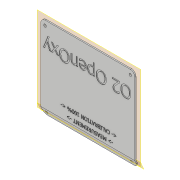
# Autodesk Inventor part: 03_Lid
Saved by Autodesk Inventor 2019.4 (Build 234330000, 330)
## iProperties
Created: 2021-06-05
Part Number: 03_Lid
Material: Generic
Document SubType Name: Modeling
Designer: diederichbenedict
Density: 1 g/cm^3
Appearance: Default
Author: diederichbenedict
Autodesk Inventor part; units mm, degrees
note: some values were not read from the file. Chosen so that the rebuilt part matches the saved one: sketch regions of "Extrusion1".
(part 1 of 2)
ref_plane "YZ Plane" through (0, 0, 0) normal (1, 0, 0) x (0, 1, 0)
ref_plane "XZ Plane" through (0, 0, 0) normal (0, 1, 0) x (-1, 0, 0)
ref_plane "XY Plane" through (0, 0, 0) normal (0, 0, 1) x (1, 0, 0)
ref_plane "Work Plane1" through (0, 0, 0) normal (0, 0, 1) x (1, 0, 0)
sketch "Sketch1" plane through (0, 0, 0) normal (0, 0, 1) x (1, 0, 0)
  ellipse E0 centre (-7.5, -84.2405) end of major axis (-7.5, -80.461) minor radius 1.5 projected
  ellipse E1 centre (-100.5, -84.2405) end of major axis (-100.5, -80.461) minor radius 1.5 projected
  ellipse E2 centre (-103, -7.7709) end of major axis (-103, -9.3506) minor radius 1.45 projected
  line L0 (-3, -61.2439) -> (-3, -12.7635) projected
  line L1 (-3, -61.2439) -> (-18, -61.2439) projected
  line L2 (-18, -90.5398) -> (-18, -61.2439) projected
  line L3 (0, -90.5398) -> (-18, -90.5398) projected
  line L4 (0, -7.7709) -> (0, -90.5398) projected
  ellipse E3 centre (-5, -7.7709) end of major axis (-5, -13.2183) minor radius 5 (0, -7.7709) -> (-5, -2.3235) ccw projected
  line L5 (-103, -2.3235) -> (-5, -2.3235) projected
  ellipse E4 centre (-103, -7.7709) end of major axis (-103, -13.2183) minor radius 5 (-103, -2.3235) -> (-108, -7.7709) ccw projected
  line L6 (-108, -90.5398) -> (-108, -7.7709) projected
  line L7 (-95, -90.5398) -> (-108, -90.5398) projected
  line L8 (-95, -61.2439) -> (-95, -90.5398) projected
  line L9 (-105, -61.2439) -> (-95, -61.2439) projected
  line L10 (-105, -12.7635) -> (-105, -61.2439) projected
  ellipse E5 centre (-103, -7.7709) end of major axis (-103, -13.2183) minor radius 5 (-105, -12.7635) -> (-98.4174, -5.5919) ccw projected
  line L11 (-9.5826, -5.5919) -> (-98.4174, -5.5919) projected
  ellipse E6 centre (-5, -7.7709) end of major axis (-5, -13.2183) minor radius 5 (-9.5826, -5.5919) -> (-3, -12.7635) ccw projected
  ellipse E7 centre (-5, -7.7709) end of major axis (-5, -9.3506) minor radius 1.45 projected
  line L12 (-18, -90.5398) -> (-95, -90.5398)
  point P0 (0, 0)
  constraints: 2 end point, 1 horizontal, 8 other
extrude "Extrusion1" add sketch "Sketch1" along normal blind 1.5 contours E0 | E1 | L1 L2 L12 L8 L9 L10 E5 L11 E6 L0 | L0 E6 L11 E5 L10 L9 L8 L7 L6 E4 L5 E3 L4 L3 L2 L1
ref_plane "Work Plane2" through (-54, -57.5226, 14.2761) normal (0, -0.3968725, 0.9178738) x (1, 0, 0)
sketch "Sketch2" plane through (-54, -57.5226, 14.2761) normal (0, -0.3968725, 0.9178738) x (1, 0, 0)
  circle A0 centre (49, -40) radius 1.45 projected
  circle A1 centre (-49, -40) radius 1.45 projected
  line L0 (-41, -35.9714) -> (-54, -35.9714) projected
  line L1 (-54, -40) -> (-54, -35.9714) projected
  arc A2 (-54, -40) -> (-49, -45) centre (-49, -40) ccw projected
  line L2 (49, -45) -> (-49, -45) projected
  arc A3 (49, -45) -> (54, -40) centre (49, -40) ccw projected
  line L3 (54, -35.9714) -> (54, -40) projected
  line L4 (54, -35.9714) -> (36, -35.9714) projected
  line L5 (36, -42) -> (36, -35.9714) projected
  line L6 (-41, -42) -> (36, -42) projected
  line L7 (-41, -35.9714) -> (-41, -42) projected
  line L8 (36, -35.9714) -> (-41, -35.9714)
  line L9 (-54, -35.9714) -> (54, -35.9714) projected
  line L10 (-54, 40) -> (-54, -35.9714) projected
  line L11 (54, -35.3761) -> (54, 40.5953) projected
  line L12 (-54, -35.9714) -> (54, -35.9714)
  line L13 (54, -35.9714) -> (54, -35.3761)
  line L14 (54, -35.3761) -> (-54, -35.3761)
  line L15 (-54, -35.3761) -> (-54, -35.9714)
  point P0 (54, 47.1327)
  constraints: 10 end point, 2 parallel, 1 collinear, 1 horizontal, 1 perpendicular
extrude "Extrusion2" add sketch "Sketch2" along normal up to surface (1.3768 mm away)
sketch "Sketch3" plane through (0, 0, 1.5) normal (0, 0, 1) x (1, 0, 0)
  ellipse E0 centre (-5, -7.7709) end of major axis (-5, -6.1911) minor radius 1.45 projected
  ellipse E1 centre (-103, -7.7709) end of major axis (-103, -6.1911) minor radius 1.45 projected
  line L0 (-108, -90.5398) -> (0, -90.5398) projected
  line L1 (0, -90.5398) -> (0, -7.7709) projected
  ellipse E2 centre (-5, -7.7709) end of major axis (-5, -13.2183) minor radius 5 (0, -7.7709) -> (-5, -2.3235) ccw projected
  line L2 (-5, -2.3235) -> (-103, -2.3235) projected
  ellipse E3 centre (-103, -7.7709) end of major axis (-103, -13.2183) minor radius 5 (-103, -2.3235) -> (-108, -7.7709) ccw projected
  line L3 (-108, -7.7709) -> (-108, -90.5398) projected
  line L4 (-3.7962, -33.7156) -> (-220.4518, -33.7156) construction
  line L5 (-220.4518, -33.7156) -> (-220.4518, 2.716) construction
  line L6 (-220.4518, 2.716) -> (-3.7962, 2.716) construction
  line L7 (-3.7962, 2.716) -> (-3.7962, -33.7156) construction
  line L8 (-24.8389, -87.8495) -> (-82.3672, -87.8495) construction
  line L9 (-82.3672, -87.8495) -> (-82.3672, -82.6215) construction
  line L10 (-82.3672, -82.6215) -> (-24.8389, -82.6215) construction
  line L11 (-24.8389, -82.6215) -> (-24.8389, -87.8495) construction
  line L12 (-20.6525, -79.3075) -> (-94.749, -79.3075) construction
  line L13 (-94.749, -79.3075) -> (-94.749, -72.5738) construction
  line L14 (-94.749, -72.5738) -> (-20.6525, -72.5738) construction
  line L15 (-20.6525, -72.5738) -> (-20.6525, -79.3075) construction
  spline S0 degree 2 poles (-14.4129, -31.9391) (-15.1575, -31.0668) (-15.9873, -28.5137) (-15.9873, -26.8754) knots 0 0 0 1 2 2 2
  spline S1 degree 2 poles (-15.9873, -26.8754) (-15.9873, -25.2798) (-15.1788, -22.6947) (-14.4129, -21.8224) knots 0 0 0 1 2 2 2
  spline S2 degree 2 poles (-14.4129, -21.8224) (-13.6044, -20.9076) (-11.4662, -20.0353) (-10.179, -20.0353) knots 0 0 0 1 2 2 2
  spline S3 degree 2 poles (-10.179, -20.0353) (-8.8492, -20.0353) (-6.7217, -20.9395) (-5.9451, -21.8224) knots 0 0 0 1 2 2 2
  spline S4 degree 2 poles (-5.9451, -21.8224) (-5.1898, -22.6947) (-4.3813, -25.2585) (-4.3813, -26.8754) knots 0 0 0 1 2 2 2
  spline S5 degree 2 poles (-4.3813, -26.8754) (-4.3813, -28.5243) (-5.2004, -31.0349) (-5.9557, -31.9391) knots 0 0 0 1 2 2 2
  spline S6 degree 2 poles (-5.9557, -31.9391) (-6.7217, -32.8114) (-8.8599, -33.7156) (-10.179, -33.7156) knots 0 0 0 1 2 2 2
  spline S7 degree 2 poles (-10.179, -33.7156) (-11.5194, -33.7156) (-13.6682, -32.7795) (-14.4129, -31.9391) knots 0 0 0 1 2 2 2
  spline S8 degree 2 poles (-14.1682, -26.8754) (-14.1682, -28.1733) (-13.6044, -30.1838) (-13.0938, -30.8434) knots 0 0 0 1 2 2 2
  spline S9 degree 2 poles (-13.0938, -30.8434) (-12.5725, -31.5242) (-11.1045, -32.205) (-10.1896, -32.205) knots 0 0 0 1 2 2 2
  spline S10 degree 2 poles (-10.1896, -32.205) (-9.2428, -32.205) (-7.8174, -31.5455) (-7.2748, -30.8434) knots 0 0 0 1 2 2 2
  spline S11 degree 2 poles (-7.2748, -30.8434) (-6.7536, -30.1732) (-6.2004, -28.152) (-6.2004, -26.8754) knots 0 0 0 1 2 2 2
  spline S12 degree 2 poles (-6.2004, -26.8754) (-6.2004, -24.2904) (-8.3705, -21.5458) (-10.1896, -21.5458) knots 0 0 0 1 2 2 2
  spline S13 degree 2 poles (-10.1896, -21.5458) (-12.0087, -21.5458) (-14.1682, -24.2904) (-14.1682, -26.8754) knots 0 0 0 1 2 2 2
  line L16 (-25.6252, -20.3118) -> (-17.5298, -20.3118)
  line L17 (-17.5298, -20.3118) -> (-17.5298, -22.1735)
  spline S14 degree 2 poles (-17.5298, -22.1735) (-18.4021, -22.9926) (-19.9552, -24.5138) (-20.6999, -25.3329) knots 0 0 0 1 2 2 2
  spline S15 degree 2 poles (-20.6999, -25.3329) (-22.1998, -26.9818) (-23.2955, -28.9605) (-23.2955, -30.0136) knots 0 0 0 1 2 2 2
  spline S16 degree 2 poles (-23.2955, -30.0136) (-23.2955, -30.5668) (-22.9551, -31.3966) (-22.6466, -31.6625) knots 0 0 0 1 2 2 2
  spline S17 degree 2 poles (-22.6466, -31.6625) (-22.3381, -31.9285) (-21.5296, -32.1944) (-21.0403, -32.1944) knots 0 0 0 1 2 2 2
  spline S18 degree 2 poles (-21.0403, -32.1944) (-20.5722, -32.1944) (-19.6148, -31.9604) (-19.1787, -31.7795) knots 0 0 0 1 2 2 2
  spline S19 degree 2 poles (-19.1787, -31.7795) (-18.8063, -31.6306) (-18.1149, -31.2051) (-17.9021, -31.0561) knots 0 0 0 1 2 2 2
  line L18 (-17.9021, -31.0561) -> (-17.8064, -31.0561)
  line L19 (-17.8064, -31.0561) -> (-17.8064, -32.9284)
  spline S20 degree 2 poles (-17.8064, -32.9284) (-18.3489, -33.1944) (-20.2956, -33.7156) (-21.168, -33.7156) knots 0 0 0 1 2 2 2
  spline S21 degree 2 poles (-21.168, -33.7156) (-23.0083, -33.7156) (-25.0827, -31.7689) (-25.0827, -30.1094) knots 0 0 0 1 2 2 2
  spline S22 degree 2 poles (-25.0827, -30.1094) (-25.0827, -29.3328) (-24.721, -28.035) (-24.4019, -27.4818) knots 0 0 0 1 2 2 2
  spline S23 degree 2 poles (-24.4019, -27.4818) (-24.0827, -26.9074) (-23.1572, -25.7797) (-22.6466, -25.2372) knots 0 0 0 1 2 2 2
  spline S24 degree 2 poles (-22.6466, -25.2372) (-21.8169, -24.333) (-19.785, -22.3969) (-19.1787, -21.8331) knots 0 0 0 1 2 2 2
  line L20 (-19.1787, -21.8331) -> (-25.6252, -21.8331)
  line L21 (-25.6252, -21.8331) -> (-25.6252, -20.3118)
  spline S25 degree 2 poles (-42.6778, -31.9391) (-43.4225, -31.0668) (-44.2523, -28.5137) (-44.2523, -26.8754) knots 0 0 0 1 2 2 2
  spline S26 degree 2 poles (-44.2523, -26.8754) (-44.2523, -25.2798) (-43.4438, -22.6947) (-42.6778, -21.8224) knots 0 0 0 1 2 2 2
  spline S27 degree 2 poles (-42.6778, -21.8224) (-41.8694, -20.9076) (-39.7311, -20.0353) (-38.4439, -20.0353) knots 0 0 0 1 2 2 2
  spline S28 degree 2 poles (-38.4439, -20.0353) (-37.1142, -20.0353) (-34.9866, -20.9395) (-34.2101, -21.8224) knots 0 0 0 1 2 2 2
  spline S29 degree 2 poles (-34.2101, -21.8224) (-33.4548, -22.6947) (-32.6463, -25.2585) (-32.6463, -26.8754) knots 0 0 0 1 2 2 2
  spline S30 degree 2 poles (-32.6463, -26.8754) (-32.6463, -28.5243) (-33.4654, -31.0349) (-34.2207, -31.9391) knots 0 0 0 1 2 2 2
  spline S31 degree 2 poles (-34.2207, -31.9391) (-34.9866, -32.8114) (-37.1248, -33.7156) (-38.4439, -33.7156) knots 0 0 0 1 2 2 2
  spline S32 degree 2 poles (-38.4439, -33.7156) (-39.7843, -33.7156) (-41.9332, -32.7795) (-42.6778, -31.9391) knots 0 0 0 1 2 2 2
  spline S33 degree 2 poles (-42.4332, -26.8754) (-42.4332, -28.1733) (-41.8694, -30.1838) (-41.3587, -30.8434) knots 0 0 0 1 2 2 2
  spline S34 degree 2 poles (-41.3587, -30.8434) (-40.8375, -31.5242) (-39.3694, -32.205) (-38.4546, -32.205) knots 0 0 0 1 2 2 2
  spline S35 degree 2 poles (-38.4546, -32.205) (-37.5078, -32.205) (-36.0823, -31.5455) (-35.5398, -30.8434) knots 0 0 0 1 2 2 2
  spline S36 degree 2 poles (-35.5398, -30.8434) (-35.0185, -30.1732) (-34.4654, -28.152) (-34.4654, -26.8754) knots 0 0 0 1 2 2 2
  spline S37 degree 2 poles (-34.4654, -26.8754) (-34.4654, -24.2904) (-36.6355, -21.5458) (-38.4546, -21.5458) knots 0 0 0 1 2 2 2
  spline S38 degree 2 poles (-38.4546, -21.5458) (-40.2737, -21.5458) (-42.4332, -24.2904) (-42.4332, -26.8754) knots 0 0 0 1 2 2 2
  spline S39 degree 2 poles (-54.2945, -25.5032) (-54.2945, -23.0352) (-51.9435, -20.1204) (-50.1457, -20.1204) knots 0 0 0 1 2 2 2
  spline S40 degree 2 poles (-50.1457, -20.1204) (-49.4116, -20.1204) (-48.284, -20.4608) (-47.6989, -20.8118) knots 0 0 0 1 2 2 2
  line L22 (-47.6989, -20.8118) -> (-47.6989, -16.6843)
  line L23 (-47.6989, -16.6843) -> (-46.0394, -16.6843)
  line L24 (-46.0394, -16.6843) -> (-46.0394, -30.1626)
  line L25 (-46.0394, -30.1626) -> (-47.6989, -30.1626)
  line L26 (-47.6989, -30.1626) -> (-47.6989, -29.1307)
  spline S41 degree 2 poles (-47.6989, -29.1307) (-48.3159, -29.6945) (-49.8265, -30.4391) (-50.7095, -30.4391) knots 0 0 0 1 2 2 2
  spline S42 degree 2 poles (-50.7095, -30.4391) (-52.4009, -30.4391) (-54.2945, -27.7584) (-54.2945, -25.5032) knots 0 0 0 1 2 2 2
  spline S43 degree 2 poles (-52.5817, -25.3117) (-52.5817, -27.0031) (-51.5073, -28.8647) (-50.3052, -28.8647) knots 0 0 0 1 2 2 2
  spline S44 degree 2 poles (-50.3052, -28.8647) (-49.6031, -28.8647) (-48.284, -28.2371) (-47.6989, -27.7478) knots 0 0 0 1 2 2 2
  line L27 (-47.6989, -27.7478) -> (-47.6989, -22.1522)
  spline S45 degree 2 poles (-47.6989, -22.1522) (-48.3479, -21.8437) (-49.2734, -21.6097) (-49.8691, -21.6097) knots 0 0 0 1 2 2 2
  spline S46 degree 2 poles (-49.8691, -21.6097) (-51.1563, -21.6097) (-52.5817, -23.5032) (-52.5817, -25.3117) knots 0 0 0 1 2 2 2
  spline S47 degree 2 poles (-60.2942, -20.0884) (-57.9326, -20.0884) (-55.337, -22.7373) (-55.337, -25.184) knots 0 0 0 1 2 2 2
  spline S48 degree 2 poles (-55.337, -25.184) (-55.337, -27.5882) (-57.8582, -30.4391) (-59.89, -30.4391) knots 0 0 0 1 2 2 2
  spline S49 degree 2 poles (-59.89, -30.4391) (-60.8049, -30.4391) (-62.2197, -29.9073) (-62.741, -29.3434) knots 0 0 0 1 2 2 2
  spline S50 degree 2 poles (-62.741, -29.3434) (-63.2729, -28.7796) (-63.8367, -27.152) (-63.8367, -25.9712) knots 0 0 0 1 2 2 2
  line L28 (-63.8367, -25.9712) -> (-63.8367, -25.067)
  line L29 (-63.8367, -25.067) -> (-57.0178, -25.067)
  spline S51 degree 2 poles (-57.0178, -25.067) (-57.0178, -23.3543) (-58.7411, -21.5352) (-60.273, -21.5352) knots 0 0 0 1 2 2 2
  spline S52 degree 2 poles (-60.273, -21.5352) (-60.8155, -21.5352) (-61.8687, -21.7799) (-62.2942, -21.9714) knots 0 0 0 1 2 2 2
  spline S53 degree 2 poles (-62.2942, -21.9714) (-62.741, -22.1841) (-63.358, -22.5564) (-63.5601, -22.7267) knots 0 0 0 1 2 2 2
  line L30 (-63.5601, -22.7267) -> (-63.6558, -22.7267)
  line L31 (-63.6558, -22.7267) -> (-63.6558, -20.9182)
  spline S54 degree 2 poles (-63.6558, -20.9182) (-63.3686, -20.8012) (-62.4963, -20.4608) (-62.1559, -20.365) knots 0 0 0 1 2 2 2
  spline S55 degree 2 poles (-62.1559, -20.365) (-61.6772, -20.2267) (-60.89, -20.0884) (-60.2942, -20.0884) knots 0 0 0 1 2 2 2
  spline S56 degree 2 poles (-62.2197, -26.3329) (-62.1984, -27.0031) (-61.9218, -27.9818) (-61.6559, -28.3116) knots 0 0 0 1 2 2 2
  spline S57 degree 2 poles (-61.6559, -28.3116) (-61.3687, -28.6839) (-60.4645, -29.0775) (-59.7943, -29.0775) knots 0 0 0 1 2 2 2
  spline S58 degree 2 poles (-59.7943, -29.0775) (-59.1347, -29.0775) (-58.2092, -28.6839) (-57.8262, -28.3009) knots 0 0 0 1 2 2 2
  spline S59 degree 2 poles (-57.8262, -28.3009) (-57.4539, -27.9073) (-57.071, -26.9605) (-57.0178, -26.3329) knots 0 0 0 1 2 2 2
  line L32 (-57.0178, -26.3329) -> (-62.2197, -26.3329)
  line L33 (-73.2512, -20.3118) -> (-71.5917, -20.3118)
  line L34 (-71.5917, -20.3118) -> (-71.5917, -25.9287)
  spline S60 degree 2 poles (-71.5917, -25.9287) (-71.5917, -26.6095) (-71.4641, -27.7797) (-71.2726, -28.1307) knots 0 0 0 1 2 2 2
  spline S61 degree 2 poles (-71.2726, -28.1307) (-71.0705, -28.503) (-70.3471, -28.8647) (-69.7301, -28.8647) knots 0 0 0 1 2 2 2
  spline S62 degree 2 poles (-69.7301, -28.8647) (-69.1131, -28.8647) (-67.8046, -28.2052) (-67.177, -27.6733) knots 0 0 0 1 2 2 2
  line L35 (-67.177, -27.6733) -> (-67.177, -20.3118)
  line L36 (-67.177, -20.3118) -> (-65.5175, -20.3118)
  line L37 (-65.5175, -20.3118) -> (-65.5175, -30.1626)
  line L38 (-65.5175, -30.1626) -> (-67.177, -30.1626)
  line L39 (-67.177, -30.1626) -> (-67.177, -29.0669)
  spline S63 degree 2 poles (-67.177, -29.0669) (-67.9216, -29.737) (-69.3578, -30.4391) (-70.1662, -30.4391) knots 0 0 0 1 2 2 2
  spline S64 degree 2 poles (-70.1662, -30.4391) (-71.613, -30.4391) (-73.2512, -28.5243) (-73.2512, -26.7052) knots 0 0 0 1 2 2 2
  line L40 (-73.2512, -26.7052) -> (-73.2512, -20.3118)
  spline S65 degree 2 poles (-84.9955, -31.9391) (-85.7402, -31.0668) (-86.5699, -28.5137) (-86.5699, -26.8754) knots 0 0 0 1 2 2 2
  spline S66 degree 2 poles (-86.5699, -26.8754) (-86.5699, -25.2798) (-85.7614, -22.6947) (-84.9955, -21.8224) knots 0 0 0 1 2 2 2
  spline S67 degree 2 poles (-84.9955, -21.8224) (-84.187, -20.9076) (-82.0488, -20.0353) (-80.7616, -20.0353) knots 0 0 0 1 2 2 2
  spline S68 degree 2 poles (-80.7616, -20.0353) (-79.4319, -20.0353) (-77.3043, -20.9395) (-76.5277, -21.8224) knots 0 0 0 1 2 2 2
  spline S69 degree 2 poles (-76.5277, -21.8224) (-75.7724, -22.6947) (-74.9639, -25.2585) (-74.9639, -26.8754) knots 0 0 0 1 2 2 2
  spline S70 degree 2 poles (-74.9639, -26.8754) (-74.9639, -28.5243) (-75.7831, -31.0349) (-76.5384, -31.9391) knots 0 0 0 1 2 2 2
  spline S71 degree 2 poles (-76.5384, -31.9391) (-77.3043, -32.8114) (-79.4425, -33.7156) (-80.7616, -33.7156) knots 0 0 0 1 2 2 2
  spline S72 degree 2 poles (-80.7616, -33.7156) (-82.102, -33.7156) (-84.2509, -32.7795) (-84.9955, -31.9391) knots 0 0 0 1 2 2 2
  spline S73 degree 2 poles (-84.7508, -26.8754) (-84.7508, -28.1733) (-84.187, -30.1838) (-83.6764, -30.8434) knots 0 0 0 1 2 2 2
  spline S74 degree 2 poles (-83.6764, -30.8434) (-83.1551, -31.5242) (-81.6871, -32.205) (-80.7723, -32.205) knots 0 0 0 1 2 2 2
  spline S75 degree 2 poles (-80.7723, -32.205) (-79.8255, -32.205) (-78.4, -31.5455) (-77.8575, -30.8434) knots 0 0 0 1 2 2 2
  spline S76 degree 2 poles (-77.8575, -30.8434) (-77.3362, -30.1732) (-76.783, -28.152) (-76.783, -26.8754) knots 0 0 0 1 2 2 2
  spline S77 degree 2 poles (-76.783, -26.8754) (-76.783, -24.2904) (-78.9532, -21.5458) (-80.7723, -21.5458) knots 0 0 0 1 2 2 2
  spline S78 degree 2 poles (-80.7723, -21.5458) (-82.5913, -21.5458) (-84.7508, -24.2904) (-84.7508, -26.8754) knots 0 0 0 1 2 2 2
  line L41 (-96.0058, -20.3118) -> (-93.9739, -20.3118)
  line L42 (-93.9739, -20.3118) -> (-91.5804, -24.0138)
  line L43 (-91.5804, -24.0138) -> (-89.123, -20.3118)
  line L44 (-89.123, -20.3118) -> (-87.2401, -20.3118)
  line L45 (-87.2401, -20.3118) -> (-90.6549, -25.1947)
  line L46 (-90.6549, -25.1947) -> (-87.272, -30.1626)
  line L47 (-87.272, -30.1626) -> (-89.3039, -30.1626)
  line L48 (-89.3039, -30.1626) -> (-91.6868, -26.4925)
  line L49 (-91.6868, -26.4925) -> (-94.1228, -30.1626)
  line L50 (-94.1228, -30.1626) -> (-96.0058, -30.1626)
  line L51 (-96.0058, -30.1626) -> (-92.6123, -25.301)
  line L52 (-92.6123, -25.301) -> (-96.0058, -20.3118)
  line L53 (-105.0267, -30.1626) -> (-99.729, -16.6843)
  line L54 (-99.729, -16.6843) -> (-97.9525, -16.6843)
  line L55 (-97.9525, -16.6843) -> (-99.7184, -20.7906)
  line L56 (-99.7184, -20.7906) -> (-96.1441, -30.1626)
  line L57 (-96.1441, -30.1626) -> (-97.9312, -30.1626)
  line L58 (-97.9312, -30.1626) -> (-100.6226, -22.8649)
  line L59 (-100.6226, -22.8649) -> (-103.3034, -30.1626)
  line L60 (-103.3034, -30.1626) -> (-105.0267, -30.1626)
  line L61 (-24.0153, -75.5057) -> (-21.1838, -76.8578)
  line L62 (-21.1838, -76.8578) -> (-21.1838, -77.1728)
  line L63 (-21.1838, -77.1728) -> (-24.0153, -78.5249)
  line L64 (-24.0153, -78.5249) -> (-24.0153, -78.0572)
  line L65 (-24.0153, -78.0572) -> (-21.8201, -77.0169)
  line L66 (-21.8201, -77.0169) -> (-24.0153, -75.9734)
  line L67 (-24.0153, -75.9734) -> (-24.0153, -75.5057)
  line L68 (-26.3058, -76.7783) -> (-24.8201, -76.7783)
  line L69 (-24.8201, -76.7783) -> (-24.8201, -77.2555)
  line L70 (-24.8201, -77.2555) -> (-26.3058, -77.2555)
  line L71 (-26.3058, -77.2555) -> (-26.3058, -76.7783)
  spline S79 degree 2 poles (-30.1585, -75.229) (-29.7767, -75.229) (-29.1309, -75.4866) (-28.8955, -75.7443) knots 0 0 0 1 2 2 2
  spline S80 degree 2 poles (-28.8955, -75.7443) (-28.6601, -75.9988) (-28.4024, -76.7624) (-28.4024, -77.2587) knots 0 0 0 1 2 2 2
  spline S81 degree 2 poles (-28.4024, -77.2587) (-28.4024, -77.7518) (-28.6537, -78.4835) (-28.8923, -78.7539) knots 0 0 0 1 2 2 2
  spline S82 degree 2 poles (-28.8923, -78.7539) (-29.1277, -79.018) (-29.7704, -79.2948) (-30.168, -79.2948) knots 0 0 0 1 2 2 2
  spline S83 degree 2 poles (-30.168, -79.2948) (-30.3653, -79.2948) (-30.7121, -79.2375) (-30.8584, -79.193) knots 0 0 0 1 2 2 2
  spline S84 degree 2 poles (-30.8584, -79.193) (-30.9857, -79.1516) (-31.2497, -79.0339) (-31.3802, -78.9639) knots 0 0 0 1 2 2 2
  line L72 (-31.3802, -78.9639) -> (-31.3802, -78.334)
  line L73 (-31.3802, -78.334) -> (-31.3388, -78.334)
  spline S85 degree 2 poles (-31.3388, -78.334) (-31.2688, -78.3976) (-31.0525, -78.5758) (-30.8966, -78.6617) knots 0 0 0 1 2 2 2
  spline S86 degree 2 poles (-30.8966, -78.6617) (-30.7471, -78.7444) (-30.3939, -78.8494) (-30.1649, -78.8494) knots 0 0 0 1 2 2 2
  spline S87 degree 2 poles (-30.1649, -78.8494) (-29.9135, -78.8494) (-29.465, -78.6426) (-29.2963, -78.4453) knots 0 0 0 1 2 2 2
  spline S88 degree 2 poles (-29.2963, -78.4453) (-29.1309, -78.2449) (-28.9464, -77.6373) (-28.9464, -77.2587) knots 0 0 0 1 2 2 2
  spline S89 degree 2 poles (-28.9464, -77.2587) (-28.9464, -76.8546) (-29.1405, -76.2724) (-29.3091, -76.072) knots 0 0 0 1 2 2 2
  spline S90 degree 2 poles (-29.3091, -76.072) (-29.4745, -75.878) (-29.9167, -75.6807) (-30.1649, -75.6807) knots 0 0 0 1 2 2 2
  spline S91 degree 2 poles (-30.1649, -75.6807) (-30.3907, -75.6807) (-30.7757, -75.7921) (-30.9252, -75.8748) knots 0 0 0 1 2 2 2
  spline S92 degree 2 poles (-30.9252, -75.8748) (-31.0684, -75.9575) (-31.2815, -76.1293) (-31.342, -76.1897) knots 0 0 0 1 2 2 2
  line L74 (-31.342, -76.1897) -> (-31.3802, -76.1897)
  line L75 (-31.3802, -76.1897) -> (-31.3802, -75.5662)
  spline S93 degree 2 poles (-31.3802, -75.5662) (-31.2497, -75.5057) (-31.0207, -75.3944) (-30.8584, -75.3435) knots 0 0 0 1 2 2 2
  spline S94 degree 2 poles (-30.8584, -75.3435) (-30.6866, -75.2862) (-30.3939, -75.229) (-30.1585, -75.229) knots 0 0 0 1 2 2 2
  line L76 (-31.4438, -75.2989) -> (-32.7672, -79.2248)
  line L77 (-32.7672, -79.2248) -> (-33.4099, -79.2248)
  line L78 (-33.4099, -79.2248) -> (-34.7333, -75.2989)
  line L79 (-34.7333, -75.2989) -> (-34.1829, -75.2989)
  line L80 (-34.1829, -75.2989) -> (-33.8266, -76.3965)
  line L81 (-33.8266, -76.3965) -> (-32.3282, -76.3965)
  line L82 (-32.3282, -76.3965) -> (-31.9719, -75.2989)
  line L83 (-31.9719, -75.2989) -> (-31.4438, -75.2989)
  line L84 (-33.6835, -76.8419) -> (-33.0758, -78.6903)
  line L85 (-33.0758, -78.6903) -> (-32.4714, -76.8419)
  line L86 (-32.4714, -76.8419) -> (-33.6835, -76.8419)
  line L87 (-37.3802, -75.2989) -> (-35.1055, -75.2989)
  line L88 (-35.1055, -75.2989) -> (-35.1055, -79.2248)
  line L89 (-35.1055, -79.2248) -> (-35.6273, -79.2248)
  line L90 (-35.6273, -79.2248) -> (-35.6273, -75.7634)
  line L91 (-35.6273, -75.7634) -> (-37.3802, -75.7634)
  line L92 (-37.3802, -75.7634) -> (-37.3802, -75.2989)
  line L93 (-39.1586, -75.2989) -> (-37.6379, -75.2989)
  line L94 (-37.6379, -75.2989) -> (-37.6379, -75.6998)
  line L95 (-37.6379, -75.6998) -> (-38.1374, -75.6998)
  line L96 (-38.1374, -75.6998) -> (-38.1374, -78.8239)
  line L97 (-38.1374, -78.8239) -> (-37.6379, -78.8239)
  line L98 (-37.6379, -78.8239) -> (-37.6379, -79.2248)
  line L99 (-37.6379, -79.2248) -> (-39.1586, -79.2248)
  line L100 (-39.1586, -79.2248) -> (-39.1586, -78.8239)
  line L101 (-39.1586, -78.8239) -> (-38.6592, -78.8239)
  line L102 (-38.6592, -78.8239) -> (-38.6592, -75.6998)
  line L103 (-38.6592, -75.6998) -> (-39.1586, -75.6998)
  line L104 (-39.1586, -75.6998) -> (-39.1586, -75.2989)
  spline S95 degree 2 poles (-42.4673, -76.5047) (-42.4673, -76.212) (-42.2446, -75.7634) (-42.06, -75.6171) knots 0 0 0 1 2 2 2
  spline S96 degree 2 poles (-42.06, -75.6171) (-41.8374, -75.4453) (-41.3315, -75.2989) (-40.9307, -75.2989) knots 0 0 0 1 2 2 2
  line L105 (-40.9307, -75.2989) -> (-39.8044, -75.2989)
  line L106 (-39.8044, -75.2989) -> (-39.8044, -79.2248)
  line L107 (-39.8044, -79.2248) -> (-40.8448, -79.2248)
  spline S97 degree 2 poles (-40.8448, -79.2248) (-41.2647, -79.2248) (-41.6846, -79.1707) (-41.8755, -79.0657) knots 0 0 0 1 2 2 2
  spline S98 degree 2 poles (-41.8755, -79.0657) (-42.0887, -78.9543) (-42.2827, -78.5885) (-42.2827, -78.3403) knots 0 0 0 1 2 2 2
  spline S99 degree 2 poles (-42.2827, -78.3403) (-42.2827, -78.0636) (-41.9901, -77.6245) (-41.7324, -77.5005) knots 0 0 0 1 2 2 2
  line L108 (-41.7324, -77.5005) -> (-41.7324, -77.4814)
  spline S100 degree 2 poles (-41.7324, -77.4814) (-42.0823, -77.3859) (-42.4673, -76.8801) (-42.4673, -76.5047) knots 0 0 0 1 2 2 2
  spline S101 degree 2 poles (-41.9232, -76.4824) (-41.9232, -76.7051) (-41.796, -76.9914) (-41.6051, -77.0932) knots 0 0 0 1 2 2 2
  spline S102 degree 2 poles (-41.6051, -77.0932) (-41.481, -77.1569) (-41.1883, -77.195) (-40.9179, -77.195) knots 0 0 0 1 2 2 2
  line L109 (-40.9179, -77.195) -> (-40.3262, -77.195)
  line L110 (-40.3262, -77.195) -> (-40.3262, -75.7443)
  line L111 (-40.3262, -75.7443) -> (-40.7493, -75.7443)
  spline S103 degree 2 poles (-40.7493, -75.7443) (-41.0929, -75.7443) (-41.4874, -75.808) (-41.6401, -75.9098) knots 0 0 0 1 2 2 2
  spline S104 degree 2 poles (-41.6401, -75.9098) (-41.7864, -76.0148) (-41.9232, -76.2756) (-41.9232, -76.4824) knots 0 0 0 1 2 2 2
  spline S105 degree 2 poles (-41.7387, -78.2672) (-41.7387, -78.4072) (-41.6433, -78.6171) (-41.5383, -78.6776) knots 0 0 0 1 2 2 2
  spline S106 degree 2 poles (-41.5383, -78.6776) (-41.411, -78.7476) (-41.1025, -78.7794) (-40.8257, -78.7794) knots 0 0 0 1 2 2 2
  line L112 (-40.8257, -78.7794) -> (-40.3262, -78.7794)
  line L113 (-40.3262, -78.7794) -> (-40.3262, -77.6309)
  line L114 (-40.3262, -77.6309) -> (-40.9179, -77.6309)
  spline S107 degree 2 poles (-40.9179, -77.6309) (-41.1629, -77.6309) (-41.3951, -77.6818) (-41.5192, -77.7613) knots 0 0 0 1 2 2 2
  spline S108 degree 2 poles (-41.5192, -77.7613) (-41.6401, -77.8377) (-41.7387, -78.0827) (-41.7387, -78.2672) knots 0 0 0 1 2 2 2
  line L115 (-46.024, -75.2989) -> (-45.3464, -75.2989)
  line L116 (-45.3464, -75.2989) -> (-44.1057, -76.861)
  line L117 (-44.1057, -76.861) -> (-43.5076, -76.861)
  line L118 (-43.5076, -76.861) -> (-43.5076, -75.2989)
  line L119 (-43.5076, -75.2989) -> (-42.9858, -75.2989)
  line L120 (-42.9858, -75.2989) -> (-42.9858, -79.2248)
  line L121 (-42.9858, -79.2248) -> (-43.9975, -79.2248)
  spline S109 degree 2 poles (-43.9975, -79.2248) (-44.3347, -79.2248) (-44.7897, -79.1516) (-44.9965, -79.018) knots 0 0 0 1 2 2 2
  spline S110 degree 2 poles (-44.9965, -79.018) (-45.2033, -78.8844) (-45.4419, -78.4676) (-45.4419, -78.159) knots 0 0 0 1 2 2 2
  spline S111 degree 2 poles (-45.4419, -78.159) (-45.4419, -77.7295) (-45.0028, -77.1473) (-44.6274, -77.0073) knots 0 0 0 1 2 2 2
  line L122 (-44.6274, -77.0073) -> (-46.024, -75.2989)
  spline S112 degree 2 poles (-44.8978, -78.1176) (-44.8978, -78.2894) (-44.7769, -78.5535) (-44.6497, -78.6394) knots 0 0 0 1 2 2 2
  spline S113 degree 2 poles (-44.6497, -78.6394) (-44.5383, -78.7126) (-44.2425, -78.773) (-44.0261, -78.773) knots 0 0 0 1 2 2 2
  line L123 (-44.0261, -78.773) -> (-43.5076, -78.773)
  line L124 (-43.5076, -78.773) -> (-43.5076, -77.2968)
  line L125 (-43.5076, -77.2968) -> (-43.9657, -77.2968)
  spline S114 degree 2 poles (-43.9657, -77.2968) (-44.1916, -77.2968) (-44.5511, -77.3764) (-44.6751, -77.5005) knots 0 0 0 1 2 2 2
  spline S115 degree 2 poles (-44.6751, -77.5005) (-44.7897, -77.6086) (-44.8978, -77.914) (-44.8978, -78.1176) knots 0 0 0 1 2 2 2
  line L126 (-45.9127, -75.2989) -> (-47.2362, -79.2248)
  line L127 (-47.2362, -79.2248) -> (-47.8788, -79.2248)
  line L128 (-47.8788, -79.2248) -> (-49.2022, -75.2989)
  line L129 (-49.2022, -75.2989) -> (-48.6519, -75.2989)
  line L130 (-48.6519, -75.2989) -> (-48.2956, -76.3965)
  line L131 (-48.2956, -76.3965) -> (-46.7971, -76.3965)
  line L132 (-46.7971, -76.3965) -> (-46.4408, -75.2989)
  line L133 (-46.4408, -75.2989) -> (-45.9127, -75.2989)
  line L134 (-48.1524, -76.8419) -> (-47.5447, -78.6903)
  line L135 (-47.5447, -78.6903) -> (-46.9403, -76.8419)
  line L136 (-46.9403, -76.8419) -> (-48.1524, -76.8419)
  line L137 (-50.4907, -75.2989) -> (-50.4907, -78.7603)
  line L138 (-50.4907, -78.7603) -> (-49.1736, -78.7603)
  line L139 (-49.1736, -78.7603) -> (-49.1736, -79.2248)
  line L140 (-49.1736, -79.2248) -> (-52.3295, -79.2248)
  line L141 (-52.3295, -79.2248) -> (-52.3295, -78.7603)
  line L142 (-52.3295, -78.7603) -> (-51.0125, -78.7603)
  line L143 (-51.0125, -78.7603) -> (-51.0125, -75.2989)
  line L144 (-51.0125, -75.2989) -> (-50.4907, -75.2989)
  line L145 (-54.0952, -75.2989) -> (-52.5745, -75.2989)
  line L146 (-52.5745, -75.2989) -> (-52.5745, -75.6998)
  line L147 (-52.5745, -75.6998) -> (-53.074, -75.6998)
  line L148 (-53.074, -75.6998) -> (-53.074, -78.8239)
  line L149 (-53.074, -78.8239) -> (-52.5745, -78.8239)
  line L150 (-52.5745, -78.8239) -> (-52.5745, -79.2248)
  line L151 (-52.5745, -79.2248) -> (-54.0952, -79.2248)
  line L152 (-54.0952, -79.2248) -> (-54.0952, -78.8239)
  line L153 (-54.0952, -78.8239) -> (-53.5957, -78.8239)
  line L154 (-53.5957, -78.8239) -> (-53.5957, -75.6998)
  line L155 (-53.5957, -75.6998) -> (-54.0952, -75.6998)
  line L156 (-54.0952, -75.6998) -> (-54.0952, -75.2989)
  spline S116 degree 2 poles (-57.5184, -78.7762) (-57.7411, -78.5153) (-57.9892, -77.7518) (-57.9892, -77.2619) knots 0 0 0 1 2 2 2
  spline S117 degree 2 poles (-57.9892, -77.2619) (-57.9892, -76.7846) (-57.7474, -76.0116) (-57.5184, -75.7507) knots 0 0 0 1 2 2 2
  spline S118 degree 2 poles (-57.5184, -75.7507) (-57.2766, -75.4771) (-56.6371, -75.2162) (-56.2522, -75.2162) knots 0 0 0 1 2 2 2
  spline S119 degree 2 poles (-56.2522, -75.2162) (-55.8545, -75.2162) (-55.2182, -75.4866) (-54.986, -75.7507) knots 0 0 0 1 2 2 2
  spline S120 degree 2 poles (-54.986, -75.7507) (-54.7601, -76.0116) (-54.5183, -76.7783) (-54.5183, -77.2619) knots 0 0 0 1 2 2 2
  spline S121 degree 2 poles (-54.5183, -77.2619) (-54.5183, -77.755) (-54.7633, -78.5058) (-54.9892, -78.7762) knots 0 0 0 1 2 2 2
  spline S122 degree 2 poles (-54.9892, -78.7762) (-55.2182, -79.0371) (-55.8577, -79.3075) (-56.2522, -79.3075) knots 0 0 0 1 2 2 2
  spline S123 degree 2 poles (-56.2522, -79.3075) (-56.653, -79.3075) (-57.2957, -79.0275) (-57.5184, -78.7762) knots 0 0 0 1 2 2 2
  spline S124 degree 2 poles (-57.4452, -77.2619) (-57.4452, -77.65) (-57.2766, -78.2513) (-57.1239, -78.4485) knots 0 0 0 1 2 2 2
  spline S125 degree 2 poles (-57.1239, -78.4485) (-56.968, -78.6521) (-56.529, -78.8557) (-56.2554, -78.8557) knots 0 0 0 1 2 2 2
  spline S126 degree 2 poles (-56.2554, -78.8557) (-55.9722, -78.8557) (-55.5459, -78.6585) (-55.3837, -78.4485) knots 0 0 0 1 2 2 2
  spline S127 degree 2 poles (-55.3837, -78.4485) (-55.2278, -78.2481) (-55.0624, -77.6436) (-55.0624, -77.2619) knots 0 0 0 1 2 2 2
  spline S128 degree 2 poles (-55.0624, -77.2619) (-55.0624, -76.4888) (-55.7114, -75.668) (-56.2554, -75.668) knots 0 0 0 1 2 2 2
  spline S129 degree 2 poles (-56.2554, -75.668) (-56.7994, -75.668) (-57.4452, -76.4888) (-57.4452, -77.2619) knots 0 0 0 1 2 2 2
  line L157 (-61.371, -75.2989) -> (-60.7857, -75.2989)
  line L158 (-60.7857, -75.2989) -> (-59.0486, -78.6839)
  line L159 (-59.0486, -78.6839) -> (-59.0486, -75.2989)
  line L160 (-59.0486, -75.2989) -> (-58.5619, -75.2989)
  line L161 (-58.5619, -75.2989) -> (-58.5619, -79.2248)
  line L162 (-58.5619, -79.2248) -> (-59.3031, -79.2248)
  line L163 (-59.3031, -79.2248) -> (-60.8843, -76.1166)
  line L164 (-60.8843, -76.1166) -> (-60.8843, -79.2248)
  line L165 (-60.8843, -79.2248) -> (-61.371, -79.2248)
  line L166 (-61.371, -79.2248) -> (-61.371, -75.2989)
  line L167 (-65.9649, -75.2989) -> (-64.0498, -75.2989)
  line L168 (-64.0498, -75.2989) -> (-64.0498, -75.6998)
  line L169 (-64.0498, -75.6998) -> (-64.7624, -75.6998)
  line L170 (-64.7624, -75.6998) -> (-64.7624, -78.3308)
  line L171 (-64.7624, -78.3308) -> (-64.0498, -78.3308)
  line L172 (-64.0498, -78.3308) -> (-64.0498, -78.6903)
  spline S130 degree 2 poles (-64.0498, -78.6903) (-64.4538, -78.6903) (-64.8356, -78.9194) (-64.861, -79.2375) knots 0 0 0 1 2 2 2
  line L173 (-64.861, -79.2375) -> (-65.2682, -79.2375)
  line L174 (-65.2682, -79.2375) -> (-65.2682, -75.6998)
  line L175 (-65.2682, -75.6998) -> (-65.9649, -75.6998)
  line L176 (-65.9649, -75.6998) -> (-65.9649, -75.2989)
  spline S131 degree 2 poles (-69.1304, -77.2619) (-69.1304, -76.2056) (-68.5164, -75.2162) (-67.877, -75.2162) knots 0 0 0 1 2 2 2
  spline S132 degree 2 poles (-67.877, -75.2162) (-67.228, -75.2162) (-66.6203, -76.2247) (-66.6203, -77.2587) knots 0 0 0 1 2 2 2
  spline S133 degree 2 poles (-66.6203, -77.2587) (-66.6203, -78.3213) (-67.2343, -79.3043) (-67.877, -79.3043) knots 0 0 0 1 2 2 2
  spline S134 degree 2 poles (-67.877, -79.3043) (-68.5228, -79.3043) (-69.1304, -78.2863) (-69.1304, -77.2619) knots 0 0 0 1 2 2 2
  spline S135 degree 2 poles (-68.456, -76.0657) (-68.5323, -76.2597) (-68.5959, -76.8578) (-68.5959, -77.2619) knots 0 0 0 1 2 2 2
  spline S136 degree 2 poles (-68.5959, -77.2619) (-68.5959, -77.6659) (-68.5323, -78.2608) (-68.4528, -78.4612) knots 0 0 0 1 2 2 2
  spline S137 degree 2 poles (-68.4528, -78.4612) (-68.3732, -78.6617) (-68.0965, -78.8685) (-67.877, -78.8685) knots 0 0 0 1 2 2 2
  spline S138 degree 2 poles (-67.877, -78.8685) (-67.6574, -78.8685) (-67.3743, -78.6617) (-67.2916, -78.4549) knots 0 0 0 1 2 2 2
  spline S139 degree 2 poles (-67.2916, -78.4549) (-67.212, -78.2544) (-67.1548, -77.6436) (-67.1548, -77.2587) knots 0 0 0 1 2 2 2
  spline S140 degree 2 poles (-67.1548, -77.2587) (-67.1548, -76.8451) (-67.2057, -76.2915) (-67.2884, -76.0752) knots 0 0 0 1 2 2 2
  spline S141 degree 2 poles (-67.2884, -76.0752) (-67.3647, -75.8716) (-67.6479, -75.6521) (-67.877, -75.6521) knots 0 0 0 1 2 2 2
  spline S142 degree 2 poles (-67.877, -75.6521) (-68.0933, -75.6521) (-68.3764, -75.8589) (-68.456, -76.0657) knots 0 0 0 1 2 2 2
  spline S143 degree 2 poles (-72.0764, -77.2619) (-72.0764, -76.2056) (-71.4624, -75.2162) (-70.8229, -75.2162) knots 0 0 0 1 2 2 2
  spline S144 degree 2 poles (-70.8229, -75.2162) (-70.1739, -75.2162) (-69.5663, -76.2247) (-69.5663, -77.2587) knots 0 0 0 1 2 2 2
  spline S145 degree 2 poles (-69.5663, -77.2587) (-69.5663, -78.3213) (-70.1803, -79.3043) (-70.8229, -79.3043) knots 0 0 0 1 2 2 2
  spline S146 degree 2 poles (-70.8229, -79.3043) (-71.4687, -79.3043) (-72.0764, -78.2863) (-72.0764, -77.2619) knots 0 0 0 1 2 2 2
  spline S147 degree 2 poles (-71.4019, -76.0657) (-71.4783, -76.2597) (-71.5419, -76.8578) (-71.5419, -77.2619) knots 0 0 0 1 2 2 2
  spline S148 degree 2 poles (-71.5419, -77.2619) (-71.5419, -77.6659) (-71.4783, -78.2608) (-71.3987, -78.4612) knots 0 0 0 1 2 2 2
  spline S149 degree 2 poles (-71.3987, -78.4612) (-71.3192, -78.6617) (-71.0424, -78.8685) (-70.8229, -78.8685) knots 0 0 0 1 2 2 2
  spline S150 degree 2 poles (-70.8229, -78.8685) (-70.6034, -78.8685) (-70.3203, -78.6617) (-70.2375, -78.4549) knots 0 0 0 1 2 2 2
  spline S151 degree 2 poles (-70.2375, -78.4549) (-70.158, -78.2544) (-70.1007, -77.6436) (-70.1007, -77.2587) knots 0 0 0 1 2 2 2
  spline S152 degree 2 poles (-70.1007, -77.2587) (-70.1007, -76.8451) (-70.1516, -76.2915) (-70.2344, -76.0752) knots 0 0 0 1 2 2 2
  spline S153 degree 2 poles (-70.2344, -76.0752) (-70.3107, -75.8716) (-70.5939, -75.6521) (-70.8229, -75.6521) knots 0 0 0 1 2 2 2
  spline S154 degree 2 poles (-70.8229, -75.6521) (-71.0392, -75.6521) (-71.3224, -75.8589) (-71.4019, -76.0657) knots 0 0 0 1 2 2 2
  spline S155 degree 2 poles (-77.2938, -76.387) (-77.2938, -75.7952) (-76.8166, -75.2226) (-76.3649, -75.2226) knots 0 0 0 1 2 2 2
  spline S156 degree 2 poles (-76.3649, -75.2226) (-75.9068, -75.2226) (-75.4359, -75.8016) (-75.4359, -76.387) knots 0 0 0 1 2 2 2
  spline S157 degree 2 poles (-75.4359, -76.387) (-75.4359, -76.9755) (-75.9163, -77.5514) (-76.3649, -77.5514) knots 0 0 0 1 2 2 2
  spline S158 degree 2 poles (-76.3649, -77.5514) (-76.8262, -77.5514) (-77.2938, -76.9723) (-77.2938, -76.387) knots 0 0 0 1 2 2 2
  spline S159 degree 2 poles (-74.4211, -78.1336) (-74.4211, -77.5418) (-73.9438, -76.9692) (-73.4921, -76.9692) knots 0 0 0 1 2 2 2
  spline S160 degree 2 poles (-73.4921, -76.9692) (-73.034, -76.9692) (-72.5631, -77.5482) (-72.5631, -78.1336) knots 0 0 0 1 2 2 2
  spline S161 degree 2 poles (-72.5631, -78.1336) (-72.5631, -78.7221) (-73.0435, -79.2979) (-73.4921, -79.2979) knots 0 0 0 1 2 2 2
  spline S162 degree 2 poles (-73.4921, -79.2979) (-73.9534, -79.2979) (-74.4211, -78.7189) (-74.4211, -78.1336) knots 0 0 0 1 2 2 2
  line L177 (-76.1772, -79.2248) -> (-74.122, -75.2989)
  line L178 (-74.122, -75.2989) -> (-73.6862, -75.2989)
  line L179 (-73.6862, -75.2989) -> (-75.7413, -79.2248)
  line L180 (-75.7413, -79.2248) -> (-76.1772, -79.2248)
  spline S163 degree 2 poles (-73.9534, -78.1336) (-73.9534, -78.5376) (-73.7657, -78.948) (-73.4953, -78.948) knots 0 0 0 1 2 2 2
  spline S164 degree 2 poles (-73.4953, -78.948) (-73.2249, -78.948) (-73.034, -78.5312) (-73.034, -78.1336) knots 0 0 0 1 2 2 2
  spline S165 degree 2 poles (-73.034, -78.1336) (-73.034, -77.7359) (-73.2121, -77.3191) (-73.4953, -77.3191) knots 0 0 0 1 2 2 2
  spline S166 degree 2 poles (-73.4953, -77.3191) (-73.7657, -77.3191) (-73.9534, -77.7359) (-73.9534, -78.1336) knots 0 0 0 1 2 2 2
  spline S167 degree 2 poles (-76.8262, -76.387) (-76.8262, -76.791) (-76.6385, -77.2014) (-76.3681, -77.2014) knots 0 0 0 1 2 2 2
  spline S168 degree 2 poles (-76.3681, -77.2014) (-76.0976, -77.2014) (-75.9068, -76.7846) (-75.9068, -76.387) knots 0 0 0 1 2 2 2
  spline S169 degree 2 poles (-75.9068, -76.387) (-75.9068, -75.9893) (-76.0849, -75.5725) (-76.3681, -75.5725) knots 0 0 0 1 2 2 2
  spline S170 degree 2 poles (-76.3681, -75.5725) (-76.6385, -75.5725) (-76.8262, -75.9893) (-76.8262, -76.387) knots 0 0 0 1 2 2 2
  line L181 (-82.6131, -75.5057) -> (-79.7817, -76.8578)
  line L182 (-79.7817, -76.8578) -> (-79.7817, -77.1728)
  line L183 (-79.7817, -77.1728) -> (-82.6131, -78.5249)
  line L184 (-82.6131, -78.5249) -> (-82.6131, -78.0572)
  line L185 (-82.6131, -78.0572) -> (-80.418, -77.0169)
  line L186 (-80.418, -77.0169) -> (-82.6131, -75.9734)
  line L187 (-82.6131, -75.9734) -> (-82.6131, -75.5057)
  line L188 (-84.9037, -76.7783) -> (-83.418, -76.7783)
  line L189 (-83.418, -76.7783) -> (-83.418, -77.2555)
  line L190 (-83.418, -77.2555) -> (-84.9037, -77.2555)
  line L191 (-84.9037, -77.2555) -> (-84.9037, -76.7783)
  line L192 (-26.5958, -85.2855) -> (-25.082, -85.2855)
  line L193 (-25.082, -85.2855) -> (-25.082, -85.7717)
  line L194 (-25.082, -85.7717) -> (-26.5958, -85.7717)
  line L195 (-26.5958, -85.7717) -> (-26.5958, -85.2855)
  line L196 (-30.2976, -85.3665) -> (-27.4127, -83.9889)
  line L197 (-27.4127, -83.9889) -> (-27.4127, -84.4654)
  line L198 (-27.4127, -84.4654) -> (-29.6493, -85.5286)
  line L199 (-29.6493, -85.5286) -> (-27.4127, -86.5886)
  line L200 (-27.4127, -86.5886) -> (-27.4127, -87.0651)
  line L201 (-27.4127, -87.0651) -> (-30.2976, -85.6874)
  line L202 (-30.2976, -85.6874) -> (-30.2976, -85.3665)
  line L203 (-36.3916, -83.7782) -> (-35.86, -83.7782)
  line L204 (-35.86, -83.7782) -> (-35.86, -87.2239)
  line L205 (-35.86, -87.2239) -> (-34.8162, -84.8803)
  line L206 (-34.8162, -84.8803) -> (-34.4921, -84.8803)
  line L207 (-34.4921, -84.8803) -> (-33.458, -87.2239)
  line L208 (-33.458, -87.2239) -> (-33.458, -83.7782)
  line L209 (-33.458, -83.7782) -> (-32.9621, -83.7782)
  line L210 (-32.9621, -83.7782) -> (-32.9621, -87.7782)
  line L211 (-32.9621, -87.7782) -> (-33.6882, -87.7782)
  line L212 (-33.6882, -87.7782) -> (-34.6866, -85.5513)
  line L213 (-34.6866, -85.5513) -> (-35.6525, -87.7782)
  line L214 (-35.6525, -87.7782) -> (-36.3916, -87.7782)
  line L215 (-36.3916, -87.7782) -> (-36.3916, -83.7782)
  line L216 (-37.202, -83.7782) -> (-37.202, -87.7782)
  line L217 (-37.202, -87.7782) -> (-39.7044, -87.7782)
  line L218 (-39.7044, -87.7782) -> (-39.7044, -87.305)
  line L219 (-39.7044, -87.305) -> (-37.7336, -87.305)
  line L220 (-37.7336, -87.305) -> (-37.7336, -86.2093)
  line L221 (-37.7336, -86.2093) -> (-39.5715, -86.2093)
  line L222 (-39.5715, -86.2093) -> (-39.5715, -85.7361)
  line L223 (-39.5715, -85.7361) -> (-37.7336, -85.7361)
  line L224 (-37.7336, -85.7361) -> (-37.7336, -84.2515)
  line L225 (-37.7336, -84.2515) -> (-39.7044, -84.2515)
  line L226 (-39.7044, -84.2515) -> (-39.7044, -83.7782)
  line L227 (-39.7044, -83.7782) -> (-37.202, -83.7782)
  line L228 (-39.8567, -83.7782) -> (-41.2052, -87.7782)
  line L229 (-41.2052, -87.7782) -> (-41.86, -87.7782)
  line L230 (-41.86, -87.7782) -> (-43.2084, -83.7782)
  line L231 (-43.2084, -83.7782) -> (-42.6477, -83.7782)
  line L232 (-42.6477, -83.7782) -> (-42.2846, -84.8965)
  line L233 (-42.2846, -84.8965) -> (-40.7579, -84.8965)
  line L234 (-40.7579, -84.8965) -> (-40.3948, -83.7782)
  line L235 (-40.3948, -83.7782) -> (-39.8567, -83.7782)
  line L236 (-42.1387, -85.3503) -> (-41.5196, -87.2336)
  line L237 (-41.5196, -87.2336) -> (-40.9037, -85.3503)
  line L238 (-40.9037, -85.3503) -> (-42.1387, -85.3503)
  spline S171 degree 2 poles (-44.7028, -83.7069) (-44.2684, -83.7069) (-43.659, -83.8884) (-43.39, -84.0181) knots 0 0 0 1 2 2 2
  line L239 (-43.39, -84.0181) -> (-43.39, -84.6858)
  line L240 (-43.39, -84.6858) -> (-43.4289, -84.6858)
  spline S172 degree 2 poles (-43.4289, -84.6858) (-43.6914, -84.4395) (-44.3559, -84.1672) (-44.6639, -84.1672) knots 0 0 0 1 2 2 2
  spline S173 degree 2 poles (-44.6639, -84.1672) (-45.1047, -84.1672) (-45.5553, -84.5335) (-45.5553, -84.8349) knots 0 0 0 1 2 2 2
  spline S174 degree 2 poles (-45.5553, -84.8349) (-45.5553, -85.0748) (-45.3187, -85.373) (-45.0626, -85.4476) knots 0 0 0 1 2 2 2
  spline S175 degree 2 poles (-45.0626, -85.4476) (-44.8778, -85.4994) (-44.5699, -85.5708) (-44.3397, -85.6291) knots 0 0 0 1 2 2 2
  spline S176 degree 2 poles (-44.3397, -85.6291) (-44.1323, -85.6842) (-43.8049, -85.8495) (-43.6785, -85.9824) knots 0 0 0 1 2 2 2
  spline S177 degree 2 poles (-43.6785, -85.9824) (-43.5553, -86.1153) (-43.4191, -86.4719) (-43.4191, -86.7053) knots 0 0 0 1 2 2 2
  spline S178 degree 2 poles (-43.4191, -86.7053) (-43.4191, -87.1915) (-44.1776, -87.8495) (-44.7644, -87.8495) knots 0 0 0 1 2 2 2
  spline S179 degree 2 poles (-44.7644, -87.8495) (-45.1015, -87.8495) (-45.6979, -87.7166) (-45.954, -87.5902) knots 0 0 0 1 2 2 2
  line L241 (-45.954, -87.5902) -> (-45.954, -86.9549)
  line L242 (-45.954, -86.9549) -> (-45.9151, -86.9549)
  spline S180 degree 2 poles (-45.9151, -86.9549) (-45.7238, -87.1299) (-45.1274, -87.3892) (-44.8, -87.3892) knots 0 0 0 1 2 2 2
  spline S181 degree 2 poles (-44.8, -87.3892) (-44.4305, -87.3892) (-43.9734, -87.0424) (-43.9734, -86.7604) knots 0 0 0 1 2 2 2
  spline S182 degree 2 poles (-43.9734, -86.7604) (-43.9734, -86.5075) (-44.2425, -86.2061) (-44.4953, -86.138) knots 0 0 0 1 2 2 2
  spline S183 degree 2 poles (-44.4953, -86.138) (-44.6639, -86.0926) (-45.1533, -85.9759) (-45.3154, -85.9273) knots 0 0 0 1 2 2 2
  spline S184 degree 2 poles (-45.3154, -85.9273) (-45.7271, -85.8009) (-46.1096, -85.292) (-46.1096, -84.9192) knots 0 0 0 1 2 2 2
  spline S185 degree 2 poles (-46.1096, -84.9192) (-46.1096, -84.6826) (-45.9183, -84.2288) (-45.7465, -84.0699) knots 0 0 0 1 2 2 2
  spline S186 degree 2 poles (-45.7465, -84.0699) (-45.5553, -83.8949) (-45.0691, -83.7069) (-44.7028, -83.7069) knots 0 0 0 1 2 2 2
  spline S187 degree 2 poles (-48.048, -83.6939) (-47.6947, -83.6939) (-47.1695, -83.8787) (-46.9848, -84.0635) knots 0 0 0 1 2 2 2
  spline S188 degree 2 poles (-46.9848, -84.0635) (-46.7741, -84.2709) (-46.6023, -84.8544) (-46.6023, -85.2823) knots 0 0 0 1 2 2 2
  line L243 (-46.6023, -85.2823) -> (-46.6023, -87.7782)
  line L244 (-46.6023, -87.7782) -> (-47.1339, -87.7782)
  line L245 (-47.1339, -87.7782) -> (-47.1339, -85.2823)
  spline S189 degree 2 poles (-47.1339, -85.2823) (-47.1339, -85.0035) (-47.2052, -84.6275) (-47.3057, -84.4751) knots 0 0 0 1 2 2 2
  spline S190 degree 2 poles (-47.3057, -84.4751) (-47.4127, -84.3131) (-47.7822, -84.1477) (-48.048, -84.1477) knots 0 0 0 1 2 2 2
  spline S191 degree 2 poles (-48.048, -84.1477) (-48.2976, -84.1477) (-48.6866, -84.3131) (-48.7935, -84.4751) knots 0 0 0 1 2 2 2
  spline S192 degree 2 poles (-48.7935, -84.4751) (-48.894, -84.6275) (-48.9653, -85.0003) (-48.9653, -85.2693) knots 0 0 0 1 2 2 2
  line L246 (-48.9653, -85.2693) -> (-48.9653, -87.7782)
  line L247 (-48.9653, -87.7782) -> (-49.4969, -87.7782)
  line L248 (-49.4969, -87.7782) -> (-49.4969, -85.2823)
  spline S193 degree 2 poles (-49.4969, -85.2823) (-49.4969, -84.8641) (-49.3284, -84.2677) (-49.1144, -84.0635) knots 0 0 0 1 2 2 2
  spline S194 degree 2 poles (-49.1144, -84.0635) (-48.9232, -83.8755) (-48.4175, -83.6939) (-48.048, -83.6939) knots 0 0 0 1 2 2 2
  line L249 (-53.3543, -83.7782) -> (-52.6639, -83.7782)
  line L250 (-52.6639, -83.7782) -> (-51.3997, -85.3698)
  line L251 (-51.3997, -85.3698) -> (-50.7903, -85.3698)
  line L252 (-50.7903, -85.3698) -> (-50.7903, -83.7782)
  line L253 (-50.7903, -83.7782) -> (-50.2587, -83.7782)
  line L254 (-50.2587, -83.7782) -> (-50.2587, -87.7782)
  line L255 (-50.2587, -87.7782) -> (-51.2895, -87.7782)
  spline S195 degree 2 poles (-51.2895, -87.7782) (-51.6331, -87.7782) (-52.0966, -87.7037) (-52.3073, -87.5675) knots 0 0 0 1 2 2 2
  spline S196 degree 2 poles (-52.3073, -87.5675) (-52.518, -87.4314) (-52.7611, -87.0067) (-52.7611, -86.6923) knots 0 0 0 1 2 2 2
  spline S197 degree 2 poles (-52.7611, -86.6923) (-52.7611, -86.2547) (-52.3138, -85.6615) (-51.9313, -85.5189) knots 0 0 0 1 2 2 2
  line L256 (-51.9313, -85.5189) -> (-53.3543, -83.7782)
  spline S198 degree 2 poles (-52.2068, -86.6502) (-52.2068, -86.8252) (-52.0836, -87.0943) (-51.954, -87.1818) knots 0 0 0 1 2 2 2
  spline S199 degree 2 poles (-51.954, -87.1818) (-51.8405, -87.2563) (-51.5391, -87.3179) (-51.3187, -87.3179) knots 0 0 0 1 2 2 2
  line L257 (-51.3187, -87.3179) -> (-50.7903, -87.3179)
  line L258 (-50.7903, -87.3179) -> (-50.7903, -85.8139)
  line L259 (-50.7903, -85.8139) -> (-51.2571, -85.8139)
  spline S200 degree 2 poles (-51.2571, -85.8139) (-51.4872, -85.8139) (-51.8535, -85.8949) (-51.9799, -86.0213) knots 0 0 0 1 2 2 2
  spline S201 degree 2 poles (-51.9799, -86.0213) (-52.0966, -86.1315) (-52.2068, -86.4427) (-52.2068, -86.6502) knots 0 0 0 1 2 2 2
  line L260 (-53.672, -83.7782) -> (-53.672, -87.7782)
  line L261 (-53.672, -87.7782) -> (-56.1744, -87.7782)
  line L262 (-56.1744, -87.7782) -> (-56.1744, -87.305)
  line L263 (-56.1744, -87.305) -> (-54.2036, -87.305)
  line L264 (-54.2036, -87.305) -> (-54.2036, -86.2093)
  line L265 (-54.2036, -86.2093) -> (-56.0415, -86.2093)
  line L266 (-56.0415, -86.2093) -> (-56.0415, -85.7361)
  line L267 (-56.0415, -85.7361) -> (-54.2036, -85.7361)
  line L268 (-54.2036, -85.7361) -> (-54.2036, -84.2515)
  line L269 (-54.2036, -84.2515) -> (-56.1744, -84.2515)
  line L270 (-56.1744, -84.2515) -> (-56.1744, -83.7782)
  line L271 (-56.1744, -83.7782) -> (-53.672, -83.7782)
  line L272 (-60.1874, -83.7782) -> (-59.6558, -83.7782)
  line L273 (-59.6558, -83.7782) -> (-59.6558, -87.2239)
  line L274 (-59.6558, -87.2239) -> (-58.612, -84.8803)
  line L275 (-58.612, -84.8803) -> (-58.2879, -84.8803)
  line L276 (-58.2879, -84.8803) -> (-57.2538, -87.2239)
  line L277 (-57.2538, -87.2239) -> (-57.2538, -83.7782)
  line L278 (-57.2538, -83.7782) -> (-56.7579, -83.7782)
  line L279 (-56.7579, -83.7782) -> (-56.7579, -87.7782)
  line L280 (-56.7579, -87.7782) -> (-57.484, -87.7782)
  line L281 (-57.484, -87.7782) -> (-58.4823, -85.5513)
  line L282 (-58.4823, -85.5513) -> (-59.4483, -87.7782)
  line L283 (-59.4483, -87.7782) -> (-60.1874, -87.7782)
  line L284 (-60.1874, -87.7782) -> (-60.1874, -83.7782)
  line L285 (-60.9977, -83.7782) -> (-60.9977, -87.7782)
  line L286 (-60.9977, -87.7782) -> (-63.5002, -87.7782)
  line L287 (-63.5002, -87.7782) -> (-63.5002, -87.305)
  line L288 (-63.5002, -87.305) -> (-61.5293, -87.305)
  line L289 (-61.5293, -87.305) -> (-61.5293, -86.2093)
  line L290 (-61.5293, -86.2093) -> (-63.3673, -86.2093)
  line L291 (-63.3673, -86.2093) -> (-63.3673, -85.7361)
  line L292 (-63.3673, -85.7361) -> (-61.5293, -85.7361)
  line L293 (-61.5293, -85.7361) -> (-61.5293, -84.2515)
  line L294 (-61.5293, -84.2515) -> (-63.5002, -84.2515)
  line L295 (-63.5002, -84.2515) -> (-63.5002, -83.7782)
  line L296 (-63.5002, -83.7782) -> (-60.9977, -83.7782)
  line L297 (-66.9459, -83.7782) -> (-66.3494, -83.7782)
  line L298 (-66.3494, -83.7782) -> (-64.5796, -87.2272)
  line L299 (-64.5796, -87.2272) -> (-64.5796, -83.7782)
  line L300 (-64.5796, -83.7782) -> (-64.0836, -83.7782)
  line L301 (-64.0836, -83.7782) -> (-64.0836, -87.7782)
  line L302 (-64.0836, -87.7782) -> (-64.8389, -87.7782)
  line L303 (-64.8389, -87.7782) -> (-66.4499, -84.6113)
  line L304 (-66.4499, -84.6113) -> (-66.4499, -87.7782)
  line L305 (-66.4499, -87.7782) -> (-66.9459, -87.7782)
  line L306 (-66.9459, -87.7782) -> (-66.9459, -83.7782)
  line L307 (-68.6898, -83.7782) -> (-68.6898, -87.305)
  line L308 (-68.6898, -87.305) -> (-67.3478, -87.305)
  line L309 (-67.3478, -87.305) -> (-67.3478, -87.7782)
  line L310 (-67.3478, -87.7782) -> (-70.5634, -87.7782)
  line L311 (-70.5634, -87.7782) -> (-70.5634, -87.305)
  line L312 (-70.5634, -87.305) -> (-69.2214, -87.305)
  line L313 (-69.2214, -87.305) -> (-69.2214, -83.7782)
  line L314 (-69.2214, -83.7782) -> (-68.6898, -83.7782)
  line L315 (-74.0383, -85.2855) -> (-72.5245, -85.2855)
  line L316 (-72.5245, -85.2855) -> (-72.5245, -85.7717)
  line L317 (-72.5245, -85.7717) -> (-74.0383, -85.7717)
  line L318 (-74.0383, -85.7717) -> (-74.0383, -85.2855)
  line L319 (-77.74, -85.3665) -> (-74.8551, -83.9889)
  line L320 (-74.8551, -83.9889) -> (-74.8551, -84.4654)
  line L321 (-74.8551, -84.4654) -> (-77.0917, -85.5286)
  line L322 (-77.0917, -85.5286) -> (-74.8551, -86.5886)
  line L323 (-74.8551, -86.5886) -> (-74.8551, -87.0651)
  line L324 (-74.8551, -87.0651) -> (-77.74, -85.6874)
  line L325 (-77.74, -85.6874) -> (-77.74, -85.3665)
  point P0 (0, 0)
  constraints: 10 other